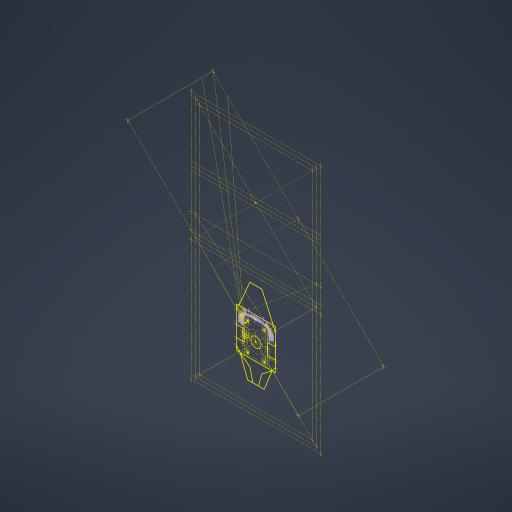
# Autodesk Inventor part: sensorcircuit
Saved by Autodesk Inventor 2023.5 (Build 275446000, 446)
## iProperties
Created: 2025-01-19
Part Number: sensorcircuit
Material: 一般
Document SubType Name: Modeling
Designer: IshiiLabHonda
Density: 1 g/cm^3
Appearance: 既定
Author: IshiiLabHonda
Autodesk Inventor part; units mm, degrees
ref_plane "YZ Plane" through (0, 0, 0) normal (1, 0, 0) x (0, 1, 0)
ref_plane "XZ Plane" through (0, 0, 0) normal (0, 1, 0) x (-1, 0, 0)
ref_plane "XY Plane" through (0, 0, 0) normal (0, 0, 1) x (1, 0, 0)
derived "chassis.ipt"
sketch "スケッチ1" plane through (0, 0, 0) normal (0, 0, 1) x (1, 0, 0)
  line L0 (-90, 90) -> (90, 90) construction
  line L1 (90, 90) -> (90, -90) construction
  line L2 (90, -90) -> (-90, -90) construction
  line L3 (-90, -90) -> (-90, 90) construction
  line L4 (-90, 90) -> (-90, 270) construction
  line L5 (-90, 270) -> (90, 270) construction
  line L6 (90, 270) -> (90, 90) construction
  line L7 (-90, 90) -> (90, -90) construction
  line L8 (90, 90) -> (-90, -90) construction
  line L9 (0, 0) -> (0, 10) construction
  line L10 (0, 0) -> (10, 0) construction
  line L11 (-90, 270) -> (90, 90) construction
  line L12 (-90, 90) -> (90, 270) construction
  line L13 (-96, 276) -> (96, 276) construction
  line L14 (96, 276) -> (96, -96) construction
  line L15 (96, -96) -> (-96, -96) construction
  line L16 (-96, -96) -> (-96, 276) construction
  line L17 (-84, 264) -> (84, 264) construction
  line L18 (84, 264) -> (84, -84) construction
  line L19 (84, -84) -> (-84, -84) construction
  line L20 (-84, -84) -> (-84, 264) construction
  line L21 (-96, 96) -> (96, 96) construction
  line L22 (-96, 84) -> (96, 84) construction
  line L23 (-63.6396, 63.6396) -> (63.6396, 190.9188) construction
  line L24 (63.6396, 190.9188) -> (190.9188, 63.6396) construction
  line L25 (190.9188, 63.6396) -> (63.6396, -63.6396) construction
  line L26 (63.6396, -63.6396) -> (-63.6396, 63.6396) construction
  line L27 (-190.9188, 190.9188) -> (-63.6396, 318.1981) construction
  line L28 (-63.6396, 318.1981) -> (63.6396, 190.9188) construction
  line L29 (-63.6396, 63.6396) -> (-190.9188, 190.9188) construction
  line L30 (-96, 120) -> (96, 120) construction
  line L31 (-96, 186) -> (96, 186) construction
  line L32 (-96, 174) -> (96, 174) construction
  line L33 (-96, 180) -> (96, 180) construction
  point P0 (-63.6396, 318.1981)
  point P1 (-90, 120)
  point P2 (90, 120)
  point P3 (0, 180)
sketch "スケッチ2" plane through (0, 0, 0) normal (0, 0, 1) x (1, 0, 0)
  line L0 (63.6396, 190.9188) -> (190.9188, 63.6396) construction
  line L1 (-63.6396, 318.1981) -> (63.6396, 190.9188) construction
  line L2 (-84, 264) -> (84, 264) construction
  line L3 (-90, 270) -> (90, 270) construction
  line L4 (90, 270) -> (90, 90) construction
  line L5 (-96, 276) -> (96, 276) construction
  line L6 (-90, 90) -> (90, 270) construction
  line L7 (-90, 270) -> (90, 90) construction
  line L8 (-63.6396, 63.6396) -> (63.6396, 190.9188) construction
  line L9 (-96, 120) -> (96, 120) construction
  line L10 (-90, 90) -> (90, 90) construction
  line L11 (-96, 96) -> (96, 96) construction
  line L12 (-96, 84) -> (96, 84) construction
  line L13 (90, -90) -> (-90, -90) construction
  line L14 (0, 0) -> (0, 10) construction
  line L15 (0, 0) -> (10, 0) construction
  line L16 (190.9188, 63.6396) -> (63.6396, -63.6396) construction
  line L17 (63.6396, -63.6396) -> (-63.6396, 63.6396) construction
  line L18 (84, -84) -> (-84, -84) construction
  line L19 (96, -96) -> (-96, -96) construction
  line L20 (-90, 90) -> (-90, 270) construction
  line L21 (-63.6396, 63.6396) -> (-190.9188, 190.9188) construction
  line L22 (-190.9188, 190.9188) -> (-63.6396, 318.1981) construction
  line L23 (96, 276) -> (96, -96) construction
  line L24 (-96, -96) -> (-96, 276) construction
  line L25 (84, 264) -> (84, -84) construction
  line L26 (-84, -84) -> (-84, 264) construction
  line L27 (90, 90) -> (90, -90) construction
  line L28 (-90, 90) -> (90, -90) construction
  line L29 (90, 90) -> (-90, -90) construction
  line L30 (-90, -90) -> (-90, 90) construction
  circle A0 centre (0, 0) radius 15 construction
  circle A1 centre (0, 0) radius 7.5 construction
  line L31 (20, 11.5) -> (28.75, 11.5) construction
  line L32 (28.75, 11.5) -> (28.75, -11.5) construction
  line L33 (28.75, -11.5) -> (20, -11.5) construction
  line L34 (20, -11.5) -> (20, 11.5) construction
  line L35 (20, 11.5) -> (18, 11.5) construction
  line L36 (18, 11.5) -> (18, -11.5) construction
  line L37 (18, -11.5) -> (20, -11.5) construction
  line L38 (18, 1.5) -> (17, 1.5) construction
  line L39 (17, -1.5) -> (18, -1.5) construction
  line L40 (-17, 24) -> (17, 24) construction
  line L41 (17, 24) -> (17, -22) construction
  line L42 (17, -22) -> (-17, -22) construction
  line L43 (-17, -22) -> (-17, 24) construction
  line L44 (-20, 11.5) -> (-18, 11.5) construction
  line L45 (-17, -1.5) -> (-18, -1.5) construction
  line L46 (-20, -11.5) -> (-20, 11.5) construction
  line L47 (-18, 11.5) -> (-18, -11.5) construction
  line L48 (-28.75, -11.5) -> (-20, -11.5) construction
  line L49 (-20, 11.5) -> (-28.75, 11.5) construction
  line L50 (-28.75, 11.5) -> (-28.75, -11.5) construction
  line L51 (-18, -11.5) -> (-20, -11.5) construction
  line L52 (-18, 1.5) -> (-17, 1.5) construction
  line L53 (-14.5, 24) -> (-14.5, -22) construction
  line L54 (14.5, 24) -> (14.5, -22) construction
  line L55 (-10.5, 24) -> (-10.5, 19) construction
  line L56 (-10.5, 19) -> (-14.5, 19) construction
  line L57 (-14.5, 24) -> (-10.5, 19) construction
  line L58 (-10.5, 24) -> (-14.5, 19) construction
  circle A2 centre (-12.5, 21.5) radius 1 construction
  line L59 (10.5, 24) -> (10.5, 19) construction
  line L60 (10.5, 19) -> (14.5, 19) construction
  line L61 (10.5, 24) -> (14.5, 19) construction
  line L62 (10.5, 19) -> (14.5, 24) construction
  circle A3 centre (12.5, 21.5) radius 1 construction
  line L63 (-14.5, -17) -> (-10.5, -17) construction
  line L64 (-10.5, -17) -> (-10.5, -22) construction
  line L65 (10.5, -22) -> (10.5, -17) construction
  line L66 (10.5, -17) -> (14.5, -17) construction
  line L67 (-14.5, -17) -> (-10.5, -22) construction
  line L68 (-10.5, -17) -> (-14.5, -22) construction
  circle A4 centre (-12.5, -19.5) radius 1 construction
  line L69 (10.5, -17) -> (14.5, -22) construction
  line L70 (14.5, -17) -> (10.5, -22) construction
  circle A5 centre (12.5, -19.5) radius 1 construction
  point P0 (90, 120)
  point P1 (-90, 120)
  point P2 (-63.6396, 318.1981)
  point P3 (-12.5, -19.5)
sketch "スケッチ3" plane through (0, 0, 0) normal (0, 0, 1) x (1, 0, 0)
  line L0 (63.6396, 190.9188) -> (190.9188, 63.6396) construction
  line L1 (-63.6396, 318.1981) -> (63.6396, 190.9188) construction
  line L2 (-84, 264) -> (84, 264) construction
  line L3 (-90, 270) -> (90, 270) construction
  line L4 (90, 270) -> (90, 90) construction
  line L5 (-96, 276) -> (96, 276) construction
  line L6 (-90, 90) -> (90, 270) construction
  line L7 (-90, 270) -> (90, 90) construction
  line L8 (-63.6396, 63.6396) -> (63.6396, 190.9188) construction
  line L9 (-96, 120) -> (96, 120) construction
  line L10 (-90, 90) -> (90, 90) construction
  line L11 (-96, 96) -> (96, 96) construction
  line L12 (-96, 84) -> (96, 84) construction
  line L13 (90, -90) -> (-90, -90) construction
  line L14 (0, 0) -> (0, 10) construction
  line L15 (0, 0) -> (10, 0) construction
  line L16 (190.9188, 63.6396) -> (63.6396, -63.6396) construction
  line L17 (63.6396, -63.6396) -> (-63.6396, 63.6396) construction
  line L18 (84, -84) -> (-84, -84) construction
  line L19 (96, -96) -> (-96, -96) construction
  line L20 (-90, 90) -> (-90, 270) construction
  line L21 (-63.6396, 63.6396) -> (-190.9188, 190.9188) construction
  line L22 (-190.9188, 190.9188) -> (-63.6396, 318.1981) construction
  line L23 (96, 276) -> (96, -96) construction
  line L24 (-96, -96) -> (-96, 276) construction
  line L25 (84, 264) -> (84, -84) construction
  line L26 (-84, -84) -> (-84, 264) construction
  line L27 (90, 90) -> (90, -90) construction
  line L28 (-90, 90) -> (90, -90) construction
  line L29 (90, 90) -> (-90, -90) construction
  line L30 (-90, -90) -> (-90, 90) construction
  line L31 (-18, 1.5) -> (-17, 1.5) construction
  line L32 (-17, -1.5) -> (-18, -1.5) construction
  line L33 (-20, 11.5) -> (-18, 11.5) construction
  line L34 (-28.75, 11.5) -> (-28.75, -11.5) construction
  line L35 (63.6396, -63.6396) -> (-63.6396, 63.6396) construction
  line L36 (84, -84) -> (-84, -84) construction
  line L37 (-90, -90) -> (-90, 90) construction
  line L38 (96, -96) -> (-96, -96) construction
  line L39 (-90, 90) -> (90, 90) construction
  line L40 (90, -90) -> (-90, -90) construction
  line L41 (90, 90) -> (-90, -90) construction
  line L42 (-90, 90) -> (90, -90) construction
  line L43 (90, 90) -> (90, -90) construction
  line L44 (-28.75, -11.5) -> (-20, -11.5) construction
  line L45 (-20, 11.5) -> (-28.75, 11.5) construction
  line L46 (-18, 11.5) -> (-18, -11.5) construction
  line L47 (-18, -11.5) -> (-20, -11.5) construction
  line L48 (0, 0) -> (0, 10) construction
  line L49 (0, 0) -> (10, 0) construction
  circle A0 centre (0, 0) radius 15 construction
  circle A1 centre (0, 0) radius 7.5
  line L50 (-14.5, 24) -> (-14.5, -22) construction
  line L51 (-17, 24) -> (17, 24) construction
  line L52 (-17, -22) -> (-17, 24) construction
  line L53 (17, -22) -> (-17, -22) construction
  line L54 (-14.5, -17) -> (-10.5, -17) construction
  circle A2 centre (-12.5, -19.5) radius 1
  line L55 (-10.5, -17) -> (-14.5, -22) construction
  line L56 (-14.5, -17) -> (-10.5, -22) construction
  line L57 (-63.6396, 318.1981) -> (63.6396, 190.9188) construction
  line L58 (-84, 264) -> (84, 264) construction
  line L59 (-90, 270) -> (90, 270) construction
  line L60 (90, 270) -> (90, 90) construction
  line L61 (-96, 276) -> (96, 276) construction
  line L62 (-90, 90) -> (90, 270) construction
  line L63 (-90, 270) -> (90, 90) construction
  line L64 (-63.6396, 63.6396) -> (63.6396, 190.9188) construction
  line L65 (-96, 120) -> (96, 120) construction
  line L66 (-96, 96) -> (96, 96) construction
  line L67 (-96, 84) -> (96, 84) construction
  line L68 (84, 264) -> (84, -84) construction
  line L69 (96, 276) -> (96, -96) construction
  line L70 (-96, -96) -> (-96, 276) construction
  line L71 (-84, -84) -> (-84, 264) construction
  line L72 (-63.6396, 63.6396) -> (-190.9188, 190.9188) construction
  line L73 (-90, 90) -> (-90, 270) construction
  line L74 (-190.9188, 190.9188) -> (-63.6396, 318.1981) construction
  line L75 (-20, -11.5) -> (-20, 11.5) construction
  line L76 (10.5, -17) -> (14.5, -17) construction
  line L77 (10.5, -22) -> (10.5, -17) construction
  circle A3 centre (12.5, -19.5) radius 1
  line L78 (10.5, -17) -> (14.5, -22) construction
  line L79 (14.5, -17) -> (10.5, -22) construction
  line L80 (-10.5, -17) -> (-10.5, -22) construction
  line L81 (63.6396, 190.9188) -> (190.9188, 63.6396) construction
  line L82 (190.9188, 63.6396) -> (63.6396, -63.6396) construction
  line L83 (20, 11.5) -> (28.75, 11.5) construction
  line L84 (28.75, 11.5) -> (28.75, -11.5) construction
  line L85 (17, -1.5) -> (18, -1.5) construction
  line L86 (18, -11.5) -> (20, -11.5) construction
  line L87 (28.75, -11.5) -> (20, -11.5) construction
  line L88 (14.5, 24) -> (14.5, -22) construction
  line L89 (17, 24) -> (17, -22) construction
  line L90 (18, 11.5) -> (18, -11.5) construction
  line L91 (20, -11.5) -> (20, 11.5) construction
  line L92 (20, 11.5) -> (18, 11.5) construction
  line L93 (18, 1.5) -> (17, 1.5) construction
  line L94 (-10.5, 24) -> (-10.5, 19) construction
  line L95 (10.5, 19) -> (14.5, 19) construction
  circle A4 centre (12.5, 21.5) radius 1
  line L96 (10.5, 24) -> (14.5, 19) construction
  line L97 (10.5, 19) -> (14.5, 24) construction
  line L98 (10.5, 24) -> (10.5, 19) construction
  line L99 (-10.5, 19) -> (-14.5, 19) construction
  circle A5 centre (-12.5, 21.5) radius 1
  line L100 (-14.5, 24) -> (-10.5, 19) construction
  line L101 (-10.5, 24) -> (-14.5, 19) construction
  line L102 (-29.25, 34.8696) -> (29.25, 34.8696)
  line L103 (29.25, 34.8696) -> (29.25, -25)
  line L104 (29.25, -25) -> (-29.25, -25)
  line L105 (-29.25, -25) -> (-29.25, 34.8696)
  line L106 (-29.25, 8.5) -> (-17, 8.5)
  line L107 (-17, 8.5) -> (-17, -8.5)
  line L108 (-17, -8.5) -> (-29.25, -8.5)
  line L109 (29.25, 8.5) -> (17, 8.5)
  line L110 (17, 8.5) -> (17, -8.5)
  line L111 (17, -8.5) -> (29.25, -8.5)
  line L112 (-13.6288, 5.5989) -> (-12.3421, -3.0559) construction
  line L113 (16.0008, 27.7912) -> (19.2148, 31.6215) construction
  line L114 (14.7835, 27.5073) -> (19.283, 32.8696) construction
  line L115 (19.7628, 23.3292) -> (14.7835, 27.5073) construction
  line L116 (19.283, 32.8696) -> (19.7628, 23.3292) construction
  line L117 (19.831, 24.5773) -> (19.2148, 31.6215) construction
  line L118 (19.831, 24.5773) -> (16.0008, 27.7912) construction
  line L119 (19.7628, 23.3292) -> (22.0609, 21.4008) construction
  line L120 (19.2148, 31.6215) -> (23.045, 28.4075) construction
  line L121 (16.0008, 27.7912) -> (23.045, 28.4075) construction
  line L122 (23.045, 28.4075) -> (19.831, 24.5773) construction
  line L123 (14.7835, 27.5073) -> (24.2623, 28.6915) construction
  line L124 (19.283, 32.8696) -> (24.2623, 28.6915) construction
  line L125 (24.2623, 28.6915) -> (19.7628, 23.3292) construction
  line L126 (22.0609, 21.4008) -> (26.5604, 26.7631) construction
  line L127 (26.5604, 26.7631) -> (24.2623, 28.6915) construction
  line L128 (-10.3326, 4.2953) -> (-8.7179, 0.3988) construction
  line L129 (-14.5076, 4.71) -> (-8.7179, 0.3988) construction
  line L130 (-13.7724, -0.2356) -> (-10.3326, 4.2953) construction
  line L131 (-14.5076, 4.71) -> (-13.7724, -0.2356) construction
  line L132 (-16.6128, 1.8696) -> (-11.5672, 2.5607) construction
  line L133 (-19.4533, 3.9748) -> (-10.3326, 4.2953) construction
  line L134 (-19.4533, 3.9748) -> (-13.7724, -0.2356) construction
  line L135 (-8.7179, 0.3988) -> (-18.718, -0.9708) construction
  line L136 (-18.718, -0.9708) -> (-14.5076, 4.71) construction
  line L137 (-20.5527, 4.5696) -> (-13.6288, 5.5989) construction
  line L138 (-18.718, -0.9708) -> (-19.4533, 3.9748) construction
  line L139 (-12.3421, -3.0559) -> (-19.266, -4.0853) construction
  line L140 (-19.266, -4.0853) -> (-20.5527, 4.5696) construction
  line L141 (-63.6396, 318.1981) -> (-16.6128, 1.8696) construction
  line L142 (19.5229, 28.0994) -> (-90, 120) construction
  line L143 (-16.6128, 1.8696) -> (-80.1088, 301.7289) construction
  line L144 (-16.6128, 1.8696) -> (-42.1821, 296.7405) construction
  line L145 (-19.5229, 28.0994) -> (90, 120) construction
  line L146 (-19.2148, 31.6215) -> (-16.0008, 27.7912) construction
  line L147 (-19.283, 32.8696) -> (-14.7835, 27.5073) construction
  line L148 (-24.2623, 28.6915) -> (-19.283, 32.8696) construction
  line L149 (-14.7835, 27.5073) -> (-24.2623, 28.6915) construction
  line L150 (-23.045, 28.4075) -> (-16.0008, 27.7912) construction
  line L151 (-23.045, 28.4075) -> (-19.2148, 31.6215) construction
  line L152 (-24.2623, 28.6915) -> (-26.5604, 26.7631) construction
  line L153 (-16.0008, 27.7912) -> (-19.831, 24.5773) construction
  line L154 (-19.2148, 31.6215) -> (-19.831, 24.5773) construction
  line L155 (-19.283, 32.8696) -> (-19.7628, 23.3292) construction
  line L156 (-14.7835, 27.5073) -> (-19.7628, 23.3292) construction
  line L157 (-19.7628, 23.3292) -> (-24.2623, 28.6915) construction
  line L158 (-26.5604, 26.7631) -> (-22.0609, 21.4008) construction
  line L159 (-22.0609, 21.4008) -> (-19.7628, 23.3292) construction
  line L160 (-19.831, 24.5773) -> (-23.045, 28.4075) construction
  line L161 (-25.6437, 34.8696) -> (-29.25, 26.6905)
  line L162 (25.6437, 34.8696) -> (29.25, 26.6905)
  line L163 (-29.25, -18.5) -> (-23.7959, -25)
  line L164 (23.7959, -25) -> (29.25, -18.5)
  circle A6 centre (-1.2011, 28.3608) radius 0.625
  circle A7 centre (-1.2011, 28.3608) radius 0.8 construction
  circle A8 centre (-1.2011, 28.3608) radius 1.5 construction
  circle A9 centre (-17.5, 33.7781) radius 1.5 construction
  circle A10 centre (-17.5, 33.7781) radius 0.8 construction
  circle A11 centre (-17.5, 33.7781) radius 0.625
  circle A12 centre (-11.4763, 34.8513) radius 1.1616
  circle A13 centre (11.4763, 34.8513) radius 1.1833
  line L165 (-13.7724, -0.2356) -> (-18.718, -0.9708) construction
  line L166 (-19.5969, -1.8597) -> (-12.673, -0.8304) construction
  line L167 (-19.0856, 1.502) -> (-14.14, 2.2372) construction
  line L168 (-18.9226, 17.4068) -> (-16.2452, -0.6032) construction
  circle A14 centre (-19, 14.8041) radius 0.625 construction
  circle A15 centre (-19, 14.8041) radius 0.8
  circle A16 centre (-19, 14.8041) radius 1.5 construction
  circle A17 centre (-15.7557, 17.2434) radius 0.625 construction
  circle A18 centre (-15.7557, 17.2434) radius 0.8
  circle A19 centre (-15.7557, 17.2434) radius 1.5 construction
  line L169 (-19.4533, 3.9748) -> (-14.5076, 4.71) construction
  line L170 (-23.7959, -25) -> (-12.5, -54.725)
  line L171 (-12.5, -54.725) -> (12.5, -54.725)
  line L172 (12.5, -54.725) -> (23.7959, -25)
  line L173 (-25.6437, 34.8696) -> (-9.098, 73.0164)
  line L174 (-9.098, 73.0164) -> (8.8244, 73.0164)
  line L175 (8.8244, 73.0164) -> (25.6437, 34.8696)
  line L176 (-23.7959, -25) -> (-9.098, -36.4234)
  line L177 (-9.098, -36.4234) -> (-4.6607, -54.725)
  line L178 (3.7452, -54.725) -> (8.8244, -36.5595)
  line L179 (8.8244, -36.5595) -> (23.7959, -25)
  point P0 (-16.6128, 1.8696)
  point P1 (-16.6128, 1.8696)
sketch "スケッチ4" plane through (0, 0, 0) normal (0, 0, 1) x (1, 0, 0)
  line L0 (-20, 11.5) -> (-28.75, 11.5) construction
  line L1 (-28.75, 11.5) -> (-28.75, -11.5) construction
  line L2 (-28.75, -11.5) -> (-20, -11.5) construction
  line L3 (20, 11.5) -> (28.75, 11.5) construction
  line L4 (18, 1.5) -> (17, 1.5) construction
  line L5 (17, -1.5) -> (18, -1.5) construction
  line L6 (18, -11.5) -> (20, -11.5) construction
  line L7 (18, 11.5) -> (18, -11.5) construction
  line L8 (14.5, 24) -> (14.5, -22) construction
  line L9 (17, 24) -> (17, -22) construction
  line L10 (20, 11.5) -> (18, 11.5) construction
  line L11 (20, -11.5) -> (20, 11.5) construction
  line L12 (28.75, -11.5) -> (20, -11.5) construction
  line L13 (28.75, 11.5) -> (28.75, -11.5) construction
  line L14 (0, 0) -> (0, 10) construction
  line L15 (0, 0) -> (10, 0) construction
  circle A0 centre (0, 0) radius 15 construction
  circle A1 centre (0, 0) radius 7.5 construction
  line L16 (-17, 24) -> (17, 24) construction
  line L17 (17, -22) -> (-17, -22) construction
  line L18 (-14.5, 24) -> (-14.5, -22) construction
  line L19 (-17, -22) -> (-17, 24) construction
  line L20 (-18, 11.5) -> (-18, -11.5) construction
  line L21 (-20, -11.5) -> (-20, 11.5) construction
  line L22 (-18, 1.5) -> (-17, 1.5) construction
  line L23 (-18, -11.5) -> (-20, -11.5) construction
  line L24 (-17, -1.5) -> (-18, -1.5) construction
  line L25 (-10.5, 19) -> (-14.5, 19) construction
  line L26 (-10.5, 24) -> (-10.5, 19) construction
  line L27 (-10.5, 24) -> (-14.5, 19) construction
  line L28 (-14.5, 24) -> (-10.5, 19) construction
  line L29 (-20, 11.5) -> (-18, 11.5) construction
  circle A2 centre (-12.5, 21.5) radius 1 construction
  line L30 (-14.5, -17) -> (-10.5, -17) construction
  circle A3 centre (-12.5, -19.5) radius 1 construction
  line L31 (-14.5, -17) -> (-10.5, -22) construction
  line L32 (-10.5, -17) -> (-14.5, -22) construction
  line L33 (-10.5, -17) -> (-10.5, -22) construction
  line L34 (10.5, -17) -> (14.5, -17) construction
  circle A4 centre (12.5, -19.5) radius 1 construction
  line L35 (10.5, -22) -> (10.5, -17) construction
  line L36 (10.5, -17) -> (14.5, -22) construction
  line L37 (14.5, -17) -> (10.5, -22) construction
  line L38 (10.5, 19) -> (14.5, 19) construction
  circle A5 centre (12.5, 21.5) radius 1 construction
  line L39 (10.5, 24) -> (14.5, 19) construction
  line L40 (10.5, 19) -> (14.5, 24) construction
  line L41 (10.5, 24) -> (10.5, 19) construction
  line L42 (0, 0) -> (0, 10) construction
  line L43 (0, 0) -> (10, 0) construction
  line L44 (0, 0) -> (0, 10) construction
  line L45 (0, 0) -> (10, 0) construction
  line L46 (10.5, -22) -> (10.5, -17) construction
  line L47 (17, -1.5) -> (18, -1.5) construction
  line L48 (18, 1.5) -> (17, 1.5) construction
  line L49 (20, -11.5) -> (20, 11.5) construction
  line L50 (18, 11.5) -> (18, -11.5) construction
  line L51 (28.75, 11.5) -> (28.75, -11.5) construction
  line L52 (-10.5, -17) -> (-10.5, -22) construction
  line L53 (10.5, 19) -> (14.5, 19) construction
  circle A6 centre (12.5, 21.5) radius 1 projected
  line L54 (-17, -1.5) -> (-18, -1.5) construction
  line L55 (14.5, 24) -> (14.5, -22) construction
  line L56 (10.5, 24) -> (14.5, 19) construction
  line L57 (10.5, 19) -> (14.5, 24) construction
  line L58 (17, 24) -> (17, -22) construction
  line L59 (10.5, 24) -> (10.5, 19) construction
  line L60 (-18, 1.5) -> (-17, 1.5) construction
  line L61 (-17, 8.5) -> (-17, -8.5) projected
  line L62 (-20, 11.5) -> (-18, 11.5) construction
  line L63 (-20, -11.5) -> (-20, 11.5) construction
  line L64 (29.25, 34.8696) -> (29.25, -25) projected
  line L65 (-29.25, -25) -> (-29.25, 34.8696) projected
  line L66 (-28.75, 11.5) -> (-28.75, -11.5) construction
  line L67 (18, -11.5) -> (20, -11.5) construction
  line L68 (10.5, -17) -> (14.5, -17) construction
  line L69 (28.75, -11.5) -> (20, -11.5) construction
  line L70 (10.5, -17) -> (14.5, -22) construction
  line L71 (20, 11.5) -> (18, 11.5) construction
  line L72 (29.25, 8.5) -> (17, 8.5) projected
  line L73 (20, 11.5) -> (28.75, 11.5) construction
  line L74 (17, 8.5) -> (17, -8.5) projected
  line L75 (-20, 11.5) -> (-28.75, 11.5) construction
  line L76 (19.283, 32.8696) -> (24.2623, 28.6915) construction
  line L77 (19.7628, 23.3292) -> (22.0609, 21.4008) construction
  line L78 (22.0609, 21.4008) -> (26.5604, 26.7631) construction
  line L79 (19.831, 24.5773) -> (19.2148, 31.6215) construction
  line L80 (16.0008, 27.7912) -> (19.2148, 31.6215) construction
  line L81 (14.7835, 27.5073) -> (19.283, 32.8696) construction
  line L82 (19.831, 24.5773) -> (16.0008, 27.7912) construction
  circle A7 centre (11.4763, 34.8513) radius 1.1833 projected
  line L83 (19.7628, 23.3292) -> (14.7835, 27.5073) construction
  line L84 (19.283, 32.8696) -> (19.7628, 23.3292) construction
  line L85 (16.0008, 27.7912) -> (23.045, 28.4075) construction
  line L86 (14.7835, 27.5073) -> (24.2623, 28.6915) construction
  line L87 (19.2148, 31.6215) -> (23.045, 28.4075) construction
  line L88 (23.045, 28.4075) -> (19.831, 24.5773) construction
  line L89 (24.2623, 28.6915) -> (19.7628, 23.3292) construction
  line L90 (26.5604, 26.7631) -> (24.2623, 28.6915) construction
  line L91 (25.6437, 34.8696) -> (29.25, 26.6905) projected
  circle A8 centre (-12.5, 21.5) radius 1 projected
  line L92 (-10.5, 19) -> (-14.5, 19) construction
  line L93 (-10.5, 24) -> (-10.5, 19) construction
  line L94 (-14.5, 24) -> (-10.5, 19) construction
  line L95 (-10.5, 24) -> (-14.5, 19) construction
  line L96 (-16.6128, 1.8696) -> (-11.5672, 2.5607) construction
  line L97 (-8.7179, 0.3988) -> (-18.718, -0.9708) construction
  line L98 (-18.718, -0.9708) -> (-19.4533, 3.9748) construction
  line L99 (-14.5076, 4.71) -> (-8.7179, 0.3988) construction
  line L100 (-14.5076, 4.71) -> (-13.7724, -0.2356) construction
  line L101 (-18.718, -0.9708) -> (-14.5076, 4.71) construction
  line L102 (-19.4533, 3.9748) -> (-13.7724, -0.2356) construction
  line L103 (-12.3421, -3.0559) -> (-19.266, -4.0853) construction
  line L104 (-19.4533, 3.9748) -> (-10.3326, 4.2953) construction
  line L105 (-10.3326, 4.2953) -> (-8.7179, 0.3988) construction
  line L106 (-13.7724, -0.2356) -> (-10.3326, 4.2953) construction
  line L107 (-13.6288, 5.5989) -> (-12.3421, -3.0559) construction
  line L108 (-20.5527, 4.5696) -> (-13.6288, 5.5989) construction
  line L109 (-19.266, -4.0853) -> (-20.5527, 4.5696) construction
  line L110 (-28.75, -11.5) -> (-20, -11.5) construction
  line L111 (-29.25, 8.5) -> (-17, 8.5) projected
  line L112 (-22.0609, 21.4008) -> (-19.7628, 23.3292) construction
  circle A9 centre (-17.5, 33.7781) radius 0.625 projected
  circle A10 centre (-17.5, 33.7781) radius 0.8 construction
  circle A11 centre (-17.5, 33.7781) radius 1.5 construction
  line L113 (-26.5604, 26.7631) -> (-22.0609, 21.4008) construction
  line L114 (-14.7835, 27.5073) -> (-19.7628, 23.3292) construction
  line L115 (-16.0008, 27.7912) -> (-19.831, 24.5773) construction
  line L116 (-14.7835, 27.5073) -> (-24.2623, 28.6915) construction
  line L117 (-23.045, 28.4075) -> (-16.0008, 27.7912) construction
  line L118 (-19.831, 24.5773) -> (-23.045, 28.4075) construction
  line L119 (-24.2623, 28.6915) -> (-26.5604, 26.7631) construction
  line L120 (-19.7628, 23.3292) -> (-24.2623, 28.6915) construction
  circle A12 centre (-11.4763, 34.8513) radius 1.1616 projected
  line L121 (-23.045, 28.4075) -> (-19.2148, 31.6215) construction
  line L122 (-19.2148, 31.6215) -> (-19.831, 24.5773) construction
  line L123 (-24.2623, 28.6915) -> (-19.283, 32.8696) construction
  line L124 (-19.283, 32.8696) -> (-19.7628, 23.3292) construction
  line L125 (-25.6437, 34.8696) -> (-29.25, 26.6905) projected
  line L126 (0, 0) -> (0, 10) construction
  line L127 (0, 0) -> (10, 0) construction
  circle A13 centre (0, 0) radius 7.5 projected
  line L128 (-14.5, -17) -> (-10.5, -17) construction
  circle A14 centre (0, 0) radius 15 construction
  circle A15 centre (12.5, -19.5) radius 1 projected
  line L129 (14.5, -17) -> (10.5, -22) construction
  circle A16 centre (-12.5, -19.5) radius 1 projected
  line L130 (-14.5, -17) -> (-10.5, -22) construction
  line L131 (17, -22) -> (-17, -22) construction
  line L132 (-29.25, 34.8696) -> (29.25, 34.8696) projected
  line L133 (23.7959, -25) -> (29.25, -18.5) projected
  line L134 (-29.25, -18.5) -> (-23.7959, -25) projected
  line L135 (29.25, -25) -> (-29.25, -25) projected
  line L136 (-17, -8.5) -> (-29.25, -8.5) projected
  line L137 (-18, -11.5) -> (-20, -11.5) construction
  line L138 (-18, 11.5) -> (-18, -11.5) construction
  circle A17 centre (-1.2011, 28.3608) radius 0.625 projected
  circle A18 centre (-1.2011, 28.3608) radius 1.5 construction
  line L139 (-19.2148, 31.6215) -> (-16.0008, 27.7912) construction
  line L140 (-19.283, 32.8696) -> (-14.7835, 27.5073) construction
  circle A19 centre (-1.2011, 28.3608) radius 0.8 construction
  line L141 (-10.5, -17) -> (-14.5, -22) construction
  line L142 (-14.5, 24) -> (-14.5, -22) construction
  line L143 (-17, -22) -> (-17, 24) construction
  line L144 (-17, 24) -> (17, 24) construction
  line L145 (17, -8.5) -> (29.25, -8.5) projected
  line L146 (-10.9787, 28.0539) -> (-12.6578, 27.2854)
  line L147 (-12.6578, 27.2854) -> (-16.5, 26.9)
  line L148 (-16.5, 26.9) -> (-19.7538, 12.1943)
  line L149 (-19.7538, 12.1943) -> (-26.6159, 14.1073)
  line L150 (-10.9787, 28.0539) -> (0, 28.0539)
  line L151 (-26.6159, 14.1073) -> (-26.0632, 22.8433)
  line L152 (-26.0632, 22.8433) -> (-21.4258, 28.4547)
  line L153 (-21.4258, 28.4547) -> (-18.0818, 29.0596)
  line L154 (-6.915, 32.35) -> (0, 33.078)
  line L155 (10.9787, 28.0539) -> (12.6578, 27.2854)
  line L156 (12.6578, 27.2854) -> (16.5, 26.9)
  line L157 (16.5, 26.9) -> (19.7538, 12.1943)
  line L158 (19.7538, 12.1943) -> (26.6159, 14.1073)
  line L159 (10.9787, 28.0539) -> (0, 28.0539)
  line L160 (26.6159, 14.1073) -> (26.0632, 22.8433)
  line L161 (26.0632, 22.8433) -> (21.4258, 28.4547)
  line L162 (21.4258, 28.4547) -> (18.0818, 29.0596)
  line L163 (6.915, 32.35) -> (0, 33.078)
  line L164 (-16.5, 34.4151) -> (-13.4256, 29.902)
  line L165 (-13.4256, 29.902) -> (-6.915, 32.35)
  line L166 (-18.0818, 29.0596) -> (-16.5, 34.4151)
  line L167 (16.5, 34.4151) -> (13.4256, 29.902)
  line L168 (18.0818, 29.0596) -> (16.5, 34.4151)
  line L169 (6.915, 32.35) -> (13.4256, 29.902)
  point P0 (-12.5, -19.5)
  point P1 (19.5229, 28.0994)
  point P2 (-16.6128, 1.8696)
  point P3 (-19.5229, 28.0994)
  constraints: 48 end point, 11 horizontal alignment, 25 other
extrude "押し出し1" add sketch "スケッチ4" against normal blind 0.6 contours A17 L150 | A17 L150 L146 L147 L148 L149 L151 L152 L153 L166 L164 L165 L154 L163 L169 L167 L168 L162 L161 L160 L158 L157 L156 L155 L159 picked at (-1.1785, 28.3633)
